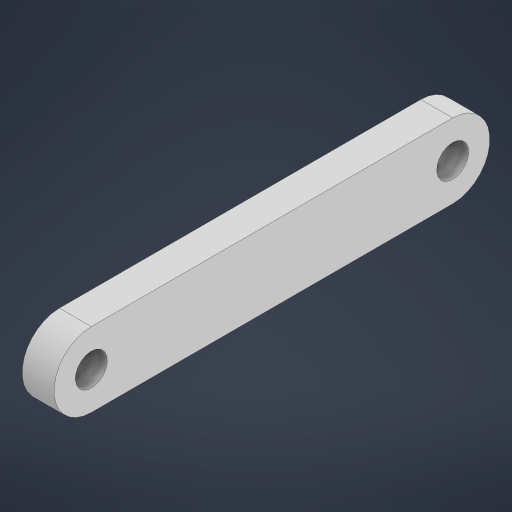
# Autodesk Inventor part: union_acr
Saved by Autodesk Inventor 2023.1 (Build 271208000, 208)
## iProperties
Created: 2022-10-23
Part Number: union_acr
Material: Generic
Document SubType Name: Modeling
Designer: amtat
Density: 1 g/cm^3
Appearance: Default
Author: amtat
Autodesk Inventor part; units mm, degrees
ref_plane "YZ Plane" through (0, 0, 0) normal (1, 0, 0) x (0, 1, 0)
ref_plane "XZ Plane" through (0, 0, 0) normal (0, 1, 0) x (-1, 0, 0)
ref_plane "XY Plane" through (0, 0, 0) normal (0, 0, 1) x (1, 0, 0)
sketch "Sketch1" plane through (0, 0, 0) normal (1, 0, 0) x (0, 1, 0)
  circle A0 centre (0, 0) radius 1.5
  arc A1 (3.5, 0) -> (-3.5, 0) centre (0, 0) ccw
  line L0 (3.5, 0) -> (3.5, -34)
  line L1 (-3.5, 0) -> (-3.5, -34)
  line L2 (-3.5, -34) -> (0, -34)
  circle A2 centre (0, -34) radius 1.5
  arc A3 (-3.5, -34) -> (3.5, -34) centre (0, -34) ccw
  dimension "d0" = 3
  dimension "d1" = 7
  dimension "d2" = 34
  dimension "d3" = 34
  dimension "d4" = 3
  constraints: 6 end point, 4 centre point, 4 coincident, 4 point on circle, 2 vertical, 1 perpendicular
  measures "d0" diameter of A0
  measures "d1" diameter of A1
  measures "d2" distance of L0.start L0.end
  measures "d3" distance of L1.start L1.end
  measures "d4" diameter of A2
extrude "Extrusion1" add sketch "Sketch1" along normal blind 3
body "Solid1"
